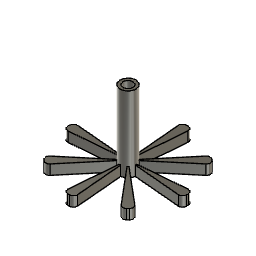
wheel base v1 (Autodesk Fusion 360 design; units mm, degrees)
Autodesk Fusion 360 part; units mm, degrees
sketch "Sketch1" plane through (0, 0, 0) normal (0, 0, 1) x (1, 0, 0)
  circle A0 centre (0, 0) radius 40
  line L0 (39.8478, 3.4862) -> (278.222, 24.3413)
  line L1 (0, 0) -> (300, 0) construction
  line L2 (39.8478, -3.4862) -> (278.222, -24.3413)
  arc A1 (299.9627, -4.7329) -> (299.9627, 4.7329) centre (0, 0) ccw
  arc A2 (299.9627, 4.7329) -> (278.222, 24.3413) centre (279.9652, 4.4174) ccw
  arc A3 (278.222, -24.3413) -> (299.9627, -4.7329) centre (279.9652, -4.4174) ccw
  line L3 (25.7115, 30.6418) -> (179.5208, 213.9446)
  line L4 (30.6418, 25.7115) -> (213.9446, 179.5208)
  arc A4 (213.9446, 179.5208) -> (215.4523, 208.759) centre (201.0888, 194.8417) ccw
  arc A5 (215.4523, 208.759) -> (208.759, 215.4523) centre (0, 0) ccw
  arc A6 (208.759, 215.4523) -> (179.5208, 213.9446) centre (194.8417, 201.0888) ccw
  line L5 (-3.4862, 39.8478) -> (-24.3413, 278.222)
  line L6 (3.4862, 39.8478) -> (24.3413, 278.222)
  arc A7 (24.3413, 278.222) -> (4.7329, 299.9627) centre (4.4174, 279.9652) ccw
  arc A8 (4.7329, 299.9627) -> (-4.7329, 299.9627) centre (0, 0) ccw
  arc A9 (-4.7329, 299.9627) -> (-24.3413, 278.222) centre (-4.4174, 279.9652) ccw
  line L7 (-30.6418, 25.7115) -> (-213.9446, 179.5208)
  line L8 (-25.7115, 30.6418) -> (-179.5208, 213.9446)
  arc A10 (-179.5208, 213.9446) -> (-208.759, 215.4523) centre (-194.8417, 201.0888) ccw
  arc A11 (-208.759, 215.4523) -> (-215.4523, 208.759) centre (0, 0) ccw
  arc A12 (-215.4523, 208.759) -> (-213.9446, 179.5208) centre (-201.0888, 194.8417) ccw
  line L9 (-39.8478, -3.4862) -> (-278.222, -24.3413)
  line L10 (-39.8478, 3.4862) -> (-278.222, 24.3413)
  arc A13 (-278.222, 24.3413) -> (-299.9627, 4.7329) centre (-279.9652, 4.4174) ccw
  arc A14 (-299.9627, 4.7329) -> (-299.9627, -4.7329) centre (0, 0) ccw
  arc A15 (-299.9627, -4.7329) -> (-278.222, -24.3413) centre (-279.9652, -4.4174) ccw
  line L11 (-25.7115, -30.6418) -> (-179.5208, -213.9446)
  line L12 (-30.6418, -25.7115) -> (-213.9446, -179.5208)
  arc A16 (-213.9446, -179.5208) -> (-215.4523, -208.759) centre (-201.0888, -194.8417) ccw
  arc A17 (-215.4523, -208.759) -> (-208.759, -215.4523) centre (0, 0) ccw
  arc A18 (-208.759, -215.4523) -> (-179.5208, -213.9446) centre (-194.8417, -201.0888) ccw
  line L13 (3.4862, -39.8478) -> (24.3413, -278.222)
  line L14 (-3.4862, -39.8478) -> (-24.3413, -278.222)
  arc A19 (-24.3413, -278.222) -> (-4.7329, -299.9627) centre (-4.4174, -279.9652) ccw
  arc A20 (-4.7329, -299.9627) -> (4.7329, -299.9627) centre (0, 0) ccw
  arc A21 (4.7329, -299.9627) -> (24.3413, -278.222) centre (4.4174, -279.9652) ccw
  line L15 (30.6418, -25.7115) -> (213.9446, -179.5208)
  line L16 (25.7115, -30.6418) -> (179.5208, -213.9446)
  arc A22 (179.5208, -213.9446) -> (208.759, -215.4523) centre (194.8417, -201.0888) ccw
  arc A23 (208.759, -215.4523) -> (215.4523, -208.759) centre (0, 0) ccw
  arc A24 (215.4523, -208.759) -> (213.9446, -179.5208) centre (201.0888, -194.8417) ccw
  point P0 (298.8584, 26.1467)
  dimension "d1" = 80
  dimension "d3" = 5
  dimension "d4" = 300
  dimension "d5" = 20
  dimension "d6" = 20
  dimension "d8" = 360
  constraint coincident A0.centre L1.start
  constraint concentric A0 A1
  constraint horizontal L1
  constraint coincident A0 L0.start
  constraint coincident A0 L2.start
  constraint coincident P0 L0
  constraint tangent L0 A2
  constraint tangent A1 A2
  constraint tangent L2 A3
  constraint tangent A1 A3
  measures "d1" diameter of A0
  measures "d3" angle of L0 L1
  measures "d4" distance of A0.centre P0
  measures "d5" radius of A2
  measures "d6" radius of A3
extrude "Extrude1" add sketch "Sketch1" along normal blind 50 contours A0 L0 L2 A1 A2 A3 | A0 L3 L4 A4 A5 A6 | A0 L15 L16 A22 A23 A24 | A0 L5 L6 A7 A8 A9 | A0 L13 L14 A19 A20 A21 | A0 L7 L8 A10 A11 A12 | A0 L11 L12 A16 A17 A18 | A0 L9 L10 A13 A14 A15 makes body 1 at (-10.4379, 119.3059, 16.6667) makes body 2 at (10.4379, -119.3059, 16.6667) makes body 3 at (-76.9813, -91.7427, 16.6667) makes body 4 at (91.7427, 76.9813, 16.6667) makes body 5 at (-91.7427, 76.9813, 16.6667) makes body 6 at (76.9813, -91.7427, 16.6667) makes body 7 at (-119.3059, -10.4379, 16.6667) makes body 8 at (119.3059, 10.4379, 16.6667)
extrude "Extrude2" add sketch "Sketch1" along normal blind 80 contours A0 bodies 1 2 3 4 5 6 7 8
extrude "Extrude3" add 1 faces at (13.1844, -1.9872, 80) along direction (0, 0, 1) blind 300 on bodies 1 bodies 1
sketch "Sketch2" plane through (0, 0, 380) normal (0, 0, 1) x (-1, 0, 0)
  circle A0 centre (0, 0) radius 40
  circle A1 centre (0, 0) radius 25
  dimension "d15" = 50
  constraint coincident A0.centre A1.centre
  measures "d15" diameter of A1
extrude "Extrude4" cut sketch "Sketch2" against normal blind 280 contours A1 bodies 1
